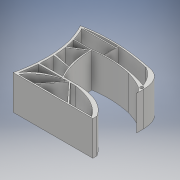
# Autodesk Inventor part: silla
Saved by Autodesk Inventor 2018 (Build 220112000, 112)
## iProperties
Created: 2018-01-12
Part Number: silla
Material: Generic
Document SubType Name: Modeling
Designer: mokuz
Density: 1 g/cm^3
Appearance: Default
Author: mokuz
Autodesk Inventor part; units mm, degrees
ref_plane "YZ Plane" through (0, 0, 0) normal (1, 0, 0) x (0, 1, 0)
ref_plane "XZ Plane" through (0, 0, 0) normal (0, 1, 0) x (-1, 0, 0)
ref_plane "XY Plane" through (0, 0, 0) normal (0, 0, 1) x (1, 0, 0)
sketch "Sketch1" plane through (0, 0, 0) normal (0, 0, 1) x (1, 0, 0)
  line L0 (161.1386, 1359.5266) -> (-238.8614, 1359.5266)
  line L1 (161.1386, 1359.5266) -> (-238.8612, 1359.5253)
  line L2 (161.1386, 1359.5266) -> (-238.8613, 1359.5262)
  line L3 (161.1386, 1359.5266) -> (-186.8113, 1142.5066)
  line L4 (248.1161, 771.1351) -> (-152.7891, 857.8121)
  line L5 (-158.5114, 459.5266) -> (400, 459.5266)
  line L6 (-32.9752, 356.2519) -> (400, 459.5266) construction
  spline S0 degree 2 poles (-213.6716, 65.4814) (-32.9752, 356.2519) (400, 459.5266) knots 1.098111 1.098111 1.098111 2 2 2
  line L7 (554.959, 459.5266) -> (223.1733, 30)
  line L8 (554.959, 459.5266) -> (955.815, 30)
  line L9 (400, 1709.5266) -> (-348.1283, 1709.5266)
  line L10 (1559.9999, 1359.5314) -> (1560, 1359.5266)
  line L11 (411.1386, 1410.8176) -> (411.1386, 1509.5266)
  spline S1 degree 2 poles (185.1086, 1363.3695) (609.3989, 1429.0606) (1059.8291, 1334.0674) knots 1.017817 1.017817 1.017817 1.648016 1.648016 1.648016
  line L12 (161.1386, 1383.5266) -> (284.9875, 1404.0635) construction
  spline S2 degree 2 poles (1488.6321, 1252.6922) (1391.0237, 1521.0798) (1159.9182, 1648.2945) knots 0 0 0 1 1 1
  line L13 (1391.0237, 1521.0798) -> (1159.9182, 1648.2945) construction
  line L14 (768.5954, 1734.2188) -> (1159.9182, 1648.2945) construction
  line L15 (1571.1386, 1017.4432) -> (1571.1386, 1177.8289) construction
  line L16 (1571.1386, 1177.8289) -> (1059.8291, 1334.0674) construction
  spline S3 degree 2 poles (1571.1386, 1017.4432) (1571.1386, 1177.8289) (1059.8291, 1334.0674) knots 1 1 1 2 2 2
  line L17 (609.3989, 1429.0606) -> (1059.8291, 1334.0674) construction
  line L18 (1571.1386, 1177.8289) -> (1560, 1593.335) construction
  line L19 (1560, 1593.335) -> (1242.767, 1672.0837) construction
  spline S4 degree 2 poles (1571.1386, 1177.8289) (1560, 1593.335) (1242.767, 1672.0837) knots 1 1 1 2 2 2
  line L20 (1087.8258, 1400.6409) -> (1488.6321, 1252.6922) construction
  spline S5 degree 2 poles (640.5331, 1411.2721) (1087.8258, 1400.6409) (1488.6321, 1252.6922) knots 1.347915 1.347915 1.347915 2 2 2
  line L21 (1488.6321, 1252.6922) -> (1391.0237, 1521.0798) construction
  line L22 (530.6033, 1416.646) -> (640.5331, 1411.2721) construction
  line L23 (640.5331, 1411.2721) -> (1087.8258, 1400.6409) construction
  line L24 (422.363, 1411.9058) -> (422.363, 1757.1534)
  line L25 (411.1386, 1685.5266) -> (-369.8693, 1685.5266)
  line L26 (-295.5796, 1541.4626) -> (-369.8693, 1685.5266) construction
  line L27 (411.1386, 1509.5266) -> (411.1386, 1685.5266)
  line L28 (400, 1709.5266) -> (400, 1758.5718)
  spline S6 degree 2 poles (422.363, 1757.1534) (768.5954, 1734.2188) (1159.9182, 1648.2945) knots 0 0 0 1 1 1
  line L29 (422.363, 1757.1534) -> (768.5954, 1734.2188) construction
  spline S7 degree 2 poles (161.1386, 1383.5266) (284.9875, 1404.0635) (411.1386, 1410.8176) knots 0 0 0 1 1 1
  spline S8 degree 2 poles (422.363, 1411.9058) (530.6033, 1416.646) (640.5331, 1411.2721) knots 0 0 0 1 1 1
  line L30 (284.9875, 1404.0635) -> (411.1386, 1410.8176) construction
  line L31 (422.363, 1411.9058) -> (530.6033, 1416.646) construction
  line L32 (161.1386, 1383.5266) -> (-246.1978, 1383.5266)
  spline S9 degree 2 poles (-246.1978, 1383.5266) (-295.5796, 1541.4626) (-369.8693, 1685.5266) knots 0 0 0 1 1 1
  line L33 (-207.3568, 1254.0684) -> (-238.8614, 1359.5266) construction
  line L34 (-246.1978, 1383.5266) -> (-295.5796, 1541.4626) construction
  line L35 (-30.322, 1016.0709) -> (-60.322, 1016.0709)
  line L36 (-280, 0) -> (-60.322, 1016.0709) construction
  line L37 (-60.322, 1016.0709) -> (-435.5436, 1709.5266) construction
  spline S10 degree 2 poles (-280, 0) (-60.322, 1016.0709) (-435.5436, 1709.5266) knots 1 1 1 2 2 2
  line L38 (1242.767, 1672.0837) -> (287.4624, 1884.9388) construction
  line L39 (287.4624, 1884.9388) -> (-443.9851, 1725.1277) construction
  spline S11 degree 2 poles (1242.767, 1672.0837) (287.4624, 1884.9388) (-443.9851, 1725.1277) knots 1 1 1 2 2 2
  line L40 (-435.5436, 1709.5266) -> (-435.5436, 1718.9513) construction
  line L41 (-435.5436, 1718.9513) -> (-443.9851, 1725.1277) construction
  spline S12 degree 2 poles (-435.5436, 1709.5266) (-435.5436, 1718.9513) (-443.9851, 1725.1277) knots 1 1 1 2 2 2
  line L42 (400, 1758.5718) -> (-26.9296, 1771.5095) construction
  line L43 (-26.9296, 1771.5095) -> (-348.1283, 1709.5266) construction
  spline S13 degree 2 poles (400, 1758.5718) (-26.9296, 1771.5095) (-348.1283, 1709.5266) knots 1 1 1 2 2 2
  line L44 (-213.6716, 65.4814) -> (-32.9752, 356.2519) construction
  line L45 (186.4589, 881.5156) -> (185.1086, 1362.7988) construction
  spline S14 degree 2 poles (397.7918, 502.1083) (186.4589, 881.5156) (185.1086, 1362.7988) knots 1.053519 1.053519 1.053519 2 2 2
  line L46 (185.1086, 1362.7988) -> (185.1086, 1363.3695)
  line L47 (185.1086, 1363.3695) -> (609.3989, 1429.0606) construction
  line L48 (-180.8353, 1108.5501) -> (163.0717, 1326.6666)
  line L49 (160.6844, 1325.1525) -> (159.3113, 1026.732) construction
  spline S15 degree 2 poles (-186.8113, 1142.5066) (-207.3568, 1254.0684) (-238.8614, 1359.5266) knots 0 0 0 1 1 1
  line L50 (-160.3886, 986.7586) -> (-180.8353, 1108.5501) construction
  line L51 (-186.8113, 1142.5066) -> (-207.3568, 1254.0684) construction
  line L52 (256.1307, 748.6567) -> (-150.7068, 816.8479)
  spline S16 degree 2 poles (-152.7891, 857.8121) (-160.3886, 986.7586) (-180.8353, 1108.5501) knots 0 0 0 1 1 1
  line L53 (-144.1812, 664.3923) -> (-150.7068, 816.8479) construction
  line L54 (-152.7891, 857.8121) -> (-160.3886, 986.7586) construction
  spline S17 degree 2 poles (160.6844, 1325.1525) (159.3113, 1026.732) (248.1161, 771.1351) knots 1.033706 1.033706 1.033706 1.621351 1.621351 1.621351
  spline S18 degree 2 poles (256.1307, 748.6567) (303.2321, 619.8647) (373.5724, 502.1083) knots 0 0 0 1 1 1
  line L55 (159.3113, 1026.732) -> (248.1161, 771.1351) construction
  line L56 (256.1307, 748.6567) -> (303.2321, 619.8647) construction
  line L57 (-155.3033, 502.1083) -> (373.5724, 502.1083)
  line L58 (303.2321, 619.8647) -> (373.5724, 502.1083) construction
  spline S19 degree 2 poles (-213.6716, 65.4814) (-174.1396, 269.1604) (-158.5114, 459.5266) knots 0 0 0 1 1 1
  spline S20 degree 2 poles (-155.3033, 502.1083) (-144.1812, 664.3923) (-150.7068, 816.8479) knots 0 0 0 1 1 1
  line L59 (-174.1396, 269.1604) -> (-158.5114, 459.5266) construction
  line L60 (-155.3033, 502.1083) -> (-144.1812, 664.3923) construction
  line L61 (-175.497, 30) -> (3.3356, 317.7714) construction
  line L62 (3.3356, 317.7714) -> (456.7489, 459.5266) construction
  spline S21 degree 2 poles (-175.497, 30) (3.3356, 317.7714) (456.7489, 459.5266) knots 1 1 1 2 2 2
  line L63 (397.7918, 502.1083) -> (718.4486, 502.1083)
  line L64 (1571.1386, 95.1334) -> (1336.4814, 481.3927) construction
  line L65 (1336.4814, 481.3927) -> (718.4486, 502.1083) construction
  spline S22 degree 2 poles (1571.1386, 95.1334) (1336.4814, 481.3927) (718.4486, 502.1083) knots 1 1 1 2 2 2
  line L66 (397.7918, 502.1083) -> (186.4589, 881.5156) construction
  line L67 (1516.7362, 30) -> (1275.4709, 372.4307) construction
  line L68 (1275.4709, 372.4307) -> (709.9179, 459.5266) construction
  spline S23 degree 2 poles (1516.7362, 30) (1275.4709, 372.4307) (709.9179, 459.5266) knots 1 1 1 2 2 2
  line L69 (-213.6716, 65.4814) -> (-174.1396, 269.1604) construction
  line L70 (1571.1386, 0) -> (1571.1386, 95.1334)
  line L71 (1571.1386, 1017.4432) -> (1571.1386, 1177.8289)
  line L72 (186.4589, 30) -> (524.6326, 459.5266)
  line L73 (589.667, 459.5266) -> (990.523, 30)
  line L74 (709.9179, 459.5266) -> (589.667, 459.5266)
  line L75 (524.6326, 459.5266) -> (456.7489, 459.5266)
  line L76 (-175.497, 30) -> (186.4589, 30)
  line L77 (223.1733, 30) -> (955.815, 30)
  line L78 (990.523, 30) -> (1516.7362, 30)
  circle A0 centre (1516.7362, 1194.4524) radius 36
  line L79 (-280, 0) -> (1571.1386, 0)
  point P0 (390.9108, 1423.4749)
  point P1 (271.3597, 1843.399)
  point P2 (-16.2977, 999.8731)
  point P3 (-67.3038, 785.2568)
  point P4 (158.4265, 834.4446)
  point P5 (-99.7467, 625.5419)
  point P6 (-135.0742, 451.6261)
  dimension "d13" = 400
  dimension "d25" = 30
  dimension "d27" = 72
  constraints: 64 end point, 10 horizontal, 5 parallel, 4 point on line, 3 vertical, 2 coincident, 2 collinear, 1 centre point, 73 other
  measures "d13" distance of L0.start L0.end
  measures "d25" distance of L35.start L35.end
  measures "d27" diameter of A0
extrude "Extrusion1" add sketch "Sketch1" along normal blind 800
body "Solid1"
